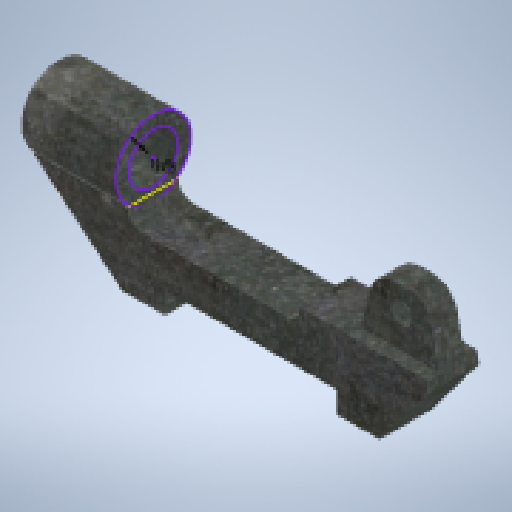
# Autodesk Inventor part: part1
Saved by Autodesk Inventor 2025.2 (Build 292293000, 293)
## iProperties
Created: 2024-12-05
Part Number: part1
Material: Stal
Document SubType Name: Modeling
Designer: Marek
Density: 7.85 g/cm^3
Appearance: Płyta
Author: Marek
Autodesk Inventor part; units mm, degrees
ref_plane "YZ Plane" through (0, 0, 0) normal (1, 0, 0) x (0, 1, 0)
ref_plane "XZ Plane" through (0, 0, 0) normal (0, 1, 0) x (-1, 0, 0)
ref_plane "XY Plane" through (0, 0, 0) normal (0, 0, 1) x (1, 0, 0)
sketch "Szkic1" plane through (0, 0, 0) normal (0, 0, 1) x (1, 0, 0)
  line L0 (0, 5) -> (0, 0)
  line L1 (0, 0) -> (10, 0)
  line L2 (0, 5) -> (-40, 5)
  line L3 (-40, 5) -> (-40, 0)
  line L4 (-40, 0) -> (-50, 0)
  line L5 (-50, 0) -> (-70.7267, 17.3918)
  line L6 (-70.7267, 17.3918) -> (-48.7267, 17.3918)
  line L7 (-48.7267, 17.3918) -> (-48.7267, 13.8918)
  line L8 (-48.7267, 13.8918) -> (-8.7267, 13.8918)
  line L9 (-8.7267, 13.8918) -> (-8.7267, 17.3918)
  line L10 (-8.7267, 17.3918) -> (2.6733, 17.3918)
  line L11 (2.6733, 17.3918) -> (5.7412, 30.6804)
  line L12 (18.2412, 30.6804) -> (5.7412, 30.6804)
  line L13 (10, 0) -> (21.0625, 14.6804)
  line L14 (18.2412, 30.6804) -> (21.0625, 14.6804)
  circle A0 centre (11.9912, 25.0804) radius 2.5
  line L15 (2.6733, 17.3918) -> (20.5844, 17.3918)
  point P0 (11.9912, 30.6804)
  dimension "d0" = 10
  dimension "d1" = 40
  dimension "d2" = 10
  dimension "d3" = 22
  dimension "d4" = 3.5
  dimension "d5" = 40
  dimension "d6" = 11.4
  dimension "d7" = 103
  dimension "d8" = 12.5
  dimension "d9" = 127
  dimension "d10" = 16
  dimension "d11" = 5
  dimension "d12" = 133
  dimension "d13" = 5
  dimension "d14" = 5.6
  constraints: 32 end point, 5 perpendicular, 4 point on line, 2 horizontal, 1 centre point, 1 midpoint, 1 vertical
  measures "d0" distance of L0.end L13.start
  measures "d1" distance of L0.start L2.end
  measures "d2" distance of L3.end L4.end
  measures "d3" distance of L5.end L7.start
  measures "d4" distance of L7.start L8.start
  measures "d5" distance of L8.start L8.end
  measures "d6" distance of L10.start L10.end
  measures "d7" angle of L11 L10
  measures "d8" distance of L11.end L12.start
  measures "d9" angle of L13 L1
  measures "d10" vertical distance of L14.end L12.start
  measures "d11" distance of L2.end L3.end
  measures "d12" angle of L13 L14
  measures "d13" diameter of A0
  measures "d14" distance of point (11.991, 30.68) A0.centre
extrude "Wyciągnięcie proste1" add sketch "Szkic1" along normal mid plane 12 contours L2 L3 L4 L5 L6 L7 L8 L9 L10 L15 L14 L13 L1 L0
extrude "Wyciągnięcie proste2" add sketch "Szkic1" along normal mid plane 6 contours L15 L11 L12 L14
fillet "Zaokrąglenie1" radius 3 1 edges at (-48.7267, 13.8918, 0)
fillet "Zaokrąglenie2" radius 3 1 edges at (-8.7267, 13.8918, 0)
fillet "Zaokrąglenie3" radius 6 1 edges at (18.2412, 30.6804, 0)
fillet "Zaokrąglenie4" radius 6 1 edges at (5.7412, 30.6804, 0)
sketch "Szkic3" plane through (-48.7267, 17.3918, 6) normal (1, 0, 0) x (0, 0, -1)
  line L0 (12, 0) -> (0, 0) projected
  circle A0 centre (6, 7) radius 8.75
  circle A1 centre (6, 7) radius 5.75
  point P0 (6, -17.3918)
  dimension "d39" = 17.5
  dimension "d40" = 11.5
  constraints: 2 centre point, 1 coincident
  measures "d39" diameter of A0
  measures "d40" diameter of A1
extrude "Wyciągnięcie proste3" add sketch "Szkic3" against normal blind 22 contours A0 L0 | L0 A0 | A1
extrude "Wyciągnięcie proste4" cut sketch "Szkic3" against normal blind 22 contours A1
